Autodesk Fusion 360 part; units mm, degrees
(part 14 of 24)
  arc A3558 (64.6096, 1.6002) -> (64.6096, 1.5494) centre (64.6096, 1.5748) ccw
  arc A3559 (65.1035, 1.8344) -> (65.1543, 1.8344) centre (65.1289, 1.8344) ccw
  line L1262 (63.0301, 1.5748) -> (62.381, 1.5748)
  arc A3560 (61.588, 2.7432) -> (61.5372, 2.7432) centre (61.5626, 2.7432) ccw
  arc A3561 (60.071, 1.8994) -> (60.1218, 1.8994) centre (60.0964, 1.8994) ccw
  arc A3562 (62.7214, 2.763) -> (62.6897, 2.7234) centre (62.7055, 2.7432) ccw
  arc A3563 (65.9384, 2.7178) -> (65.9384, 2.7686) centre (65.9384, 2.7432) ccw
  line L1263 (64.6096, 1.5748) -> (64.8693, 1.5748)
  arc A3564 (65.5814, 1.8344) -> (65.841, 1.5748) centre (65.841, 1.8344) ccw
  arc A3565 (66.1727, 2.4836) -> (66.2235, 2.4836) centre (66.1981, 2.4836) ccw
  arc A3566 (60.1218, 2.7432) -> (60.071, 2.7432) centre (60.0964, 2.7432) ccw
  arc A3567 (65.6068, 1.8344) -> (65.556, 1.8344) centre (65.5814, 1.8344) ccw
  arc A3568 (64.8693, 1.6002) -> (64.8693, 1.5494) centre (64.8693, 1.5748) ccw
  arc A3569 (65.7112, 2.0616) -> (65.5814, 1.8344) centre (65.8451, 1.8344) ccw
  arc A3570 (66.96, 2.7432) -> (66.9092, 2.7432) centre (66.9346, 2.7432) ccw
  arc A3571 (66.6101, 2.7686) -> (66.6101, 2.7178) centre (66.6101, 2.7432) ccw
  line L1264 (67.2592, 2.7432) -> (66.6101, 2.7432)
  arc A3572 (65.841, 1.5494) -> (65.841, 1.6002) centre (65.841, 1.5748) ccw
  arc A3573 (62.6802, 1.5748) -> (62.731, 1.5748) centre (62.7056, 1.5748) ccw
  line L1265 (63.0301, 2.4836) -> (62.7056, 2.7432)
  arc A3574 (61.8712, 2.4637) -> (61.903, 2.5034) centre (61.8871, 2.4835) ccw
  arc A3575 (67.2592, 2.7178) -> (67.2592, 2.7686) centre (67.2592, 2.7432) ccw
  arc A3576 (65.1035, 2.4836) -> (65.1543, 2.4836) centre (65.1289, 2.4836) ccw
  arc A3577 (64.8693, 1.5494) -> (64.8693, 1.6002) centre (64.8693, 1.5748) ccw
  line L1266 (62.7056, 2.7432) -> (62.7056, 1.5748)
  arc A3578 (65.841, 1.6002) -> (65.841, 1.5494) centre (65.841, 1.5748) ccw
  arc A3579 (66.9092, 1.5748) -> (66.96, 1.5748) centre (66.9346, 1.5748) ccw
  arc A3580 (59.4473, 1.8994) -> (60.0964, 1.8994) centre (59.7719, 1.8994) ccw
  line L1267 (64.1731, 2.4836) -> (63.8486, 2.7432)
  arc A3581 (65.7241, 2.0397) -> (65.6983, 2.0835) centre (65.7112, 2.0616) ccw
  line L1268 (61.8871, 1.5748) -> (61.238, 1.5748)
  arc A3582 (65.6991, 2.0839) -> (65.7234, 2.0393) centre (65.7113, 2.0616) ccw
  line L1269 (63.8486, 2.7432) -> (63.8486, 1.5748)
  arc A3583 (62.731, 2.7432) -> (62.6802, 2.7432) centre (62.7056, 2.7432) ccw
  arc A3584 (65.841, 1.5748) -> (66.2305, 1.7371) centre (65.841, 2.1233) ccw
  arc A3585 (60.1218, 1.8994) -> (60.071, 1.8994) centre (60.0964, 1.8994) ccw
  arc A3586 (64.6096, 2.7686) -> (64.6096, 2.7178) centre (64.6096, 2.7432) ccw
  line L1270 (66.9346, 1.5748) -> (66.9346, 2.7432)
  arc A3587 (64.8693, 2.7686) -> (64.8693, 2.7178) centre (64.8693, 2.7432) ccw
  arc A3588 (63.874, 2.7432) -> (63.8232, 2.7432) centre (63.8486, 2.7432) ccw
  arc A3589 (59.4727, 1.8994) -> (59.4219, 1.8994) centre (59.4473, 1.8994) ccw
  arc A3590 (39.4305, 29.7091) -> (39.7238, 29.8306) centre (39.5772, 29.7698) ccw
  line L1271 (38.7475, 29.511) -> (39.41, 30.1735)
  line L1272 (52.2496, 23.4133) -> (52.3555, 23.3074)
  line L1273 (53.2211, 22.9489) -> (53.34, 22.9489)
  arc A3591 (53.1962, 22.7921) -> (53.2459, 23.1057) centre (53.2211, 22.9489) ccw
  arc A3592 (52.6878, 22.9182) -> (52.8319, 23.2011) centre (52.7599, 23.0597) ccw
  arc A3593 (47.9089, 22.8537) -> (47.9089, 22.5361) centre (47.9089, 22.6949) ccw
  line L1274 (28.1196, 27.3867) -> (27.813, 27.6933)
  arc A3594 (53.34, 22.7902) -> (53.34, 23.1077) centre (53.34, 22.9489) ccw
  arc A3595 (47.1478, 22.8514) -> (47.3723, 23.0759) centre (47.2601, 22.9636) ccw
  line L1275 (45.5255, 24.4221) -> (46.4947, 24.4221)
  line L1276 (52.9861, 22.9861) -> (53.2211, 22.9489)
  arc A3596 (52.4488, 23.4359) -> (52.2621, 23.179) centre (52.3555, 23.3075) ccw
  arc A3597 (52.2432, 23.1952) -> (52.4677, 23.4197) centre (52.3555, 23.3075) ccw
  arc A3598 (53.0109, 23.1429) -> (52.9613, 22.8293) centre (52.9861, 22.9861) ccw
  arc A3599 (47.3208, 23.1103) -> (47.1993, 22.817) centre (47.2601, 22.9636) ccw
  arc A3600 (47.8481, 22.5482) -> (47.9696, 22.8416) centre (47.9089, 22.6949) ccw
  arc A3601 (39.6894, 29.8821) -> (39.4649, 29.6576) centre (39.5772, 29.7699) ccw
  arc A3602 (52.62, 23.3091) -> (52.4758, 23.0262) centre (52.5479, 23.1677) ccw
  arc A3603 (29.3289, 27.6923) -> (29.3289, 28.0098) centre (29.3289, 27.8511) ccw
  arc A3604 (27.9717, 28.7366) -> (27.6542, 28.7366) centre (27.813, 28.7366) ccw
  arc A3605 (40.3906, 29.3851) -> (40.3906, 29.0676) centre (40.3906, 29.2264) ccw
  line L1277 (49.26, 22.9637) -> (49.53, 23.2337)
  line L1278 (46.4947, 24.4221) -> (46.4947, 24.1091)
  arc A3606 (52.3619, 23.301) -> (52.1373, 23.5255) centre (52.2496, 23.4133) ccw
  arc A3607 (52.8089, 23.2106) -> (52.7108, 22.9086) centre (52.7599, 23.0596) ccw
  arc A3608 (49.8608, 23.1103) -> (49.7393, 22.817) centre (49.8, 22.9637) ccw
  arc A3609 (29.0911, 28.0098) -> (29.0911, 27.6923) centre (29.0911, 27.8511) ccw
  line L1279 (39.9298, 29.4172) -> (40.3906, 29.2263)
  arc A3610 (39.5566, 30.2343) -> (39.2633, 30.1128) centre (39.41, 30.1736) ccw
  line L1280 (29.3289, 27.8511) -> (29.21, 27.8511)
  arc A3611 (50.4489, 22.8537) -> (50.4489, 22.5361) centre (50.4489, 22.6949) ccw
  arc A3612 (52.937, 22.8351) -> (53.0352, 23.1371) centre (52.9861, 22.9861) ccw
  arc A3613 (38.2666, 29.4837) -> (38.3881, 29.1903) centre (38.3274, 29.337) ccw
  line L1281 (46.7634, 23.4602) -> (47.26, 22.9637)
  line L1282 (51.8, 22.9637) -> (52.2496, 23.4133)
  line L1283 (52.7599, 23.0596) -> (52.9861, 22.9861)
  arc A3614 (51.0904, 22.8416) -> (51.2119, 22.5482) centre (51.1512, 22.6949) ccw
  line L1284 (52.5479, 23.1676) -> (52.7599, 23.0596)
  line L1285 (52.3555, 23.3074) -> (52.5479, 23.1676)
  arc A3615 (52.4546, 23.0392) -> (52.6412, 23.296) centre (52.5479, 23.1676) ccw
  line L1286 (40.5107, 29.2263) -> (45.1661, 24.571)
  line L1287 (49.8, 22.9637) -> (50.4489, 22.6949)
  arc A3616 (45.4647, 24.2754) -> (45.5862, 24.5688) centre (45.5255, 24.4221) ccw
  arc A3617 (46.6414, 24.1698) -> (46.348, 24.0483) centre (46.4947, 24.1091) ccw
  line L1288 (40.3906, 29.2263) -> (40.5107, 29.2263)
  arc A3618 (29.3538, 28.0079) -> (29.3041, 27.6943) centre (29.329, 27.8511) ccw
  line L1289 (53.34, 22.9489) -> (53.34, 25.4)
  arc A3619 (52.3619, 23.5255) -> (52.1373, 23.301) centre (52.2496, 23.4132) ccw
  arc A3620 (51.6877, 23.0759) -> (51.9122, 22.8514) centre (51.7999, 22.9637) ccw
  arc A3621 (49.1477, 23.0759) -> (49.3722, 22.8514) centre (49.26, 22.9637) ccw
  arc A3622 (40.5107, 29.0676) -> (40.5107, 29.3851) centre (40.5107, 29.2264) ccw
  arc A3623 (46.8757, 23.5725) -> (46.6512, 23.348) centre (46.7635, 23.4603) ccw
  arc A3624 (53.2211, 23.1077) -> (53.2211, 22.7902) centre (53.2211, 22.9489) ccw
  line L1290 (47.26, 22.9637) -> (47.9089, 22.6949)
  arc A3625 (45.2268, 24.7176) -> (45.1053, 24.4243) centre (45.166, 24.5709) ccw
  arc A3626 (51.8607, 22.817) -> (51.7392, 23.1103) centre (51.7999, 22.9637) ccw
  arc A3627 (48.6111, 22.5361) -> (48.6111, 22.8537) centre (48.6111, 22.6949) ccw
  arc A3628 (46.4947, 24.2633) -> (46.4947, 24.5809) centre (46.4947, 24.4221) ccw
  arc A3629 (45.5255, 24.5809) -> (45.5255, 24.2633) centre (45.5255, 24.4221) ccw
  arc A3630 (49.3207, 22.817) -> (49.1992, 23.1103) centre (49.26, 22.9637) ccw
  line L1291 (46.4947, 24.1091) -> (46.7634, 23.4602)
  arc A3631 (48.5504, 22.8416) -> (48.6719, 22.5482) centre (48.6112, 22.6949) ccw
  arc A3632 (45.0538, 24.4587) -> (45.2783, 24.6832) centre (45.166, 24.571) ccw
  line L1292 (48.6111, 22.6949) -> (49.26, 22.9637)
  arc A3633 (53.4988, 25.4) -> (53.1813, 25.4) centre (53.3401, 25.4) ccw
  line L1293 (49.53, 23.2337) -> (49.8, 22.9637)
  arc A3634 (53.1813, 22.9489) -> (53.4988, 22.9489) centre (53.3401, 22.9489) ccw
  line L1294 (54.7406, 23.8801) -> (54.8141, 24.1063)
  arc A3635 (53.4987, 25.4) -> (53.1812, 25.4) centre (53.34, 25.4) ccw
  arc A3636 (54.761, 23.5748) -> (54.5041, 23.7614) centre (54.6326, 23.6681) ccw
  arc A3637 (54.8513, 25.2413) -> (54.8513, 25.5588) centre (54.8513, 25.4001) ccw
  line L1295 (50.4489, 22.6949) -> (51.1511, 22.6949)
  arc A3638 (51.1511, 22.5361) -> (51.1511, 22.8537) centre (51.1511, 22.6949) ccw
  line L1296 (51.1511, 22.6949) -> (51.8, 22.9637)
  arc A3639 (46.336, 24.1091) -> (46.6534, 24.1091) centre (46.4947, 24.1091) ccw
  line L1297 (54.6326, 23.6681) -> (54.7406, 23.8801)
  line L1298 (54.1321, 23.1676) -> (54.3245, 23.3074)
  arc A3640 (53.34, 23.1077) -> (53.34, 22.7902) centre (53.34, 22.9489) ccw
  arc A3641 (46.6168, 23.3995) -> (46.9101, 23.521) centre (46.7634, 23.4603) ccw
  arc A3642 (54.6631, 26.6446) -> (54.9651, 26.7428) centre (54.8141, 26.6937) ccw
  line L1299 (54.4928, 23.4757) -> (54.6326, 23.6681)
  line L1300 (53.4589, 22.9489) -> (53.6939, 22.9861)
  arc A3643 (54.882, 23.808) -> (54.5991, 23.9521) centre (54.7405, 23.8801) ccw
  line L1301 (47.9089, 22.6949) -> (48.6111, 22.6949)
  arc A3644 (50.3881, 22.5482) -> (50.5096, 22.8416) centre (50.4489, 22.6949) ccw
  arc A3645 (54.2042, 23.0262) -> (54.06, 23.3091) centre (54.1321, 23.1677) ccw
  arc A3646 (49.6878, 22.8514) -> (49.9123, 23.0759) centre (49.8, 22.9637) ccw
  arc A3647 (55.0081, 24.3164) -> (54.6945, 24.3661) centre (54.8513, 24.3413) ccw
  arc A3648 (54.8513, 25.2412) -> (54.8513, 25.5587) centre (54.8513, 25.4) ccw
  line L1302 (53.34, 25.4) -> (54.8513, 25.4)
  arc A3649 (54.6945, 26.4339) -> (55.0081, 26.4836) centre (54.8513, 26.4588) ccw
  arc A3650 (46.6534, 24.4221) -> (46.336, 24.4221) centre (46.4947, 24.4221) ccw
  arc A3651 (49.6423, 23.1214) -> (49.4177, 23.3459) centre (49.53, 23.2336) ccw
  line L1303 (54.8141, 26.6937) -> (54.7406, 26.9199)
  arc A3652 (53.4341, 23.1057) -> (53.4838, 22.7921) centre (53.459, 22.9489) ccw
  arc A3653 (54.6925, 24.3413) -> (55.01, 24.3413) centre (54.8513, 24.3413) ccw
  line L1304 (54.8513, 25.4) -> (54.8513, 26.4587)
  arc A3654 (53.7187, 22.8293) -> (53.6691, 23.1429) centre (53.6939, 22.9861) ccw
  line L1305 (54.8513, 26.4587) -> (54.8141, 26.6937)
  arc A3655 (53.4589, 22.7902) -> (53.4589, 23.1077) centre (53.4589, 22.9489) ccw
  arc A3656 (54.5041, 27.0386) -> (54.761, 27.2252) centre (54.6326, 27.1319) ccw
  line L1306 (53.34, 25.4) -> (53.34, 22.9489)
  arc A3657 (54.9651, 24.0572) -> (54.6631, 24.1554) centre (54.8141, 24.1063) ccw
  arc A3658 (53.1813, 25.4) -> (53.4988, 25.4) centre (53.3401, 25.4) ccw
  arc A3659 (55.01, 26.4587) -> (54.6925, 26.4587) centre (54.8513, 26.4587) ccw
  arc A3660 (53.9692, 22.9086) -> (53.8711, 23.2106) centre (53.9201, 23.0596) ccw
  arc A3661 (49.6423, 23.3459) -> (49.4177, 23.1214) centre (49.53, 23.2336) ccw
  line L1307 (54.8513, 25.4) -> (53.34, 25.4)
  line L1308 (54.8141, 24.1063) -> (54.8513, 24.3413)
  line L1309 (54.4928, 27.3243) -> (54.3245, 27.4926)
  arc A3662 (53.34, 25.2412) -> (53.34, 25.5587) centre (53.34, 25.4) ccw
  line L1310 (54.7406, 26.9199) -> (54.6326, 27.1319)
  arc A3663 (54.9709, 26.7185) -> (54.6573, 26.6689) centre (54.8141, 26.6937) ccw
  arc A3664 (53.34, 25.5588) -> (53.34, 25.2413) centre (53.34, 25.4001) ccw
  line L1311 (54.8513, 24.3413) -> (54.8513, 25.4)
  line L1312 (45.1661, 24.571) -> (45.5255, 24.4221)
  arc A3665 (55.01, 25.4) -> (54.6925, 25.4) centre (54.8513, 25.4) ccw
  arc A3666 (40.623, 29.3386) -> (40.3985, 29.114) centre (40.5108, 29.2263) ccw
  arc A3667 (53.6448, 23.1371) -> (53.743, 22.8351) centre (53.6939, 22.9861) ccw
  arc A3668 (54.6212, 27.4177) -> (54.3643, 27.231) centre (54.4928, 27.3244) ccw
  arc A3669 (54.4179, 23.179) -> (54.2312, 23.4359) centre (54.3246, 23.3075) ccw
  arc A3670 (54.605, 23.3634) -> (54.3805, 23.5879) centre (54.4928, 23.4757) ccw
  arc A3671 (54.3643, 23.569) -> (54.6212, 23.3823) centre (54.4928, 23.4757) ccw
  arc A3672 (54.5896, 23.9291) -> (54.8916, 23.831) centre (54.7406, 23.8801) ccw
  arc A3673 (53.8481, 23.2011) -> (53.9922, 22.9182) centre (53.9202, 23.0597) ccw
  arc A3674 (52.9613, 27.9707) -> (53.0109, 27.6571) centre (52.9861, 27.8139) ccw
  arc A3675 (53.1812, 25.4) -> (53.4987, 25.4) centre (53.34, 25.4) ccw
  arc A3676 (54.6573, 24.1311) -> (54.9709, 24.0815) centre (54.8141, 24.1063) ccw
  arc A3677 (54.774, 27.204) -> (54.4911, 27.0598) centre (54.6326, 27.1319) ccw
  arc A3678 (54.5991, 26.8479) -> (54.882, 26.992) centre (54.7405, 26.92) ccw
  arc A3679 (53.34, 25.5587) -> (53.34, 25.2412) centre (53.34, 25.4) ccw
  arc A3680 (54.0388, 23.296) -> (54.2254, 23.0392) centre (54.1321, 23.1676) ccw
  line L1313 (53.34, 22.9489) -> (53.4589, 22.9489)
  arc A3681 (54.4911, 23.7402) -> (54.774, 23.596) centre (54.6326, 23.6681) ccw
  arc A3682 (54.8916, 26.969) -> (54.5896, 26.8709) centre (54.7406, 26.92) ccw
  arc A3683 (47.2781, 34.3097) -> (47.1566, 34.0163) centre (47.2174, 34.163) ccw
  arc A3684 (47.5767, 33.8423) -> (47.6982, 34.1357) centre (47.6375, 33.989) ccw
  arc A3685 (53.743, 27.9649) -> (53.6448, 27.6629) centre (53.6939, 27.8139) ccw
  arc A3686 (47.8467, 33.5552) -> (48.0712, 33.7797) centre (47.959, 33.6675) ccw
  arc A3687 (54.06, 27.4909) -> (54.2042, 27.7738) centre (54.1321, 27.6324) ccw
  line L1314 (52.9861, 27.8139) -> (52.7599, 27.7404)
  arc A3688 (53.34, 25.5587) -> (53.34, 25.2412) centre (53.34, 25.4) ccw
  arc A3689 (53.6691, 27.6571) -> (53.7187, 27.9707) centre (53.6939, 27.8139) ccw
  arc A3690 (53.0352, 27.6629) -> (52.937, 27.9649) centre (52.9861, 27.8139) ccw
  line L1315 (54.3245, 23.3074) -> (54.4928, 23.4757)
  arc A3691 (53.4988, 27.8511) -> (53.1813, 27.8511) centre (53.3401, 27.8511) ccw
  arc A3692 (51.6567, 29.7452) -> (51.8812, 29.9697) centre (51.769, 29.8575) ccw
  line L1316 (54.3245, 27.4926) -> (54.1321, 27.6324)
  arc A3693 (52.1017, 29.4374) -> (51.7842, 29.4374) centre (51.943, 29.4374) ccw
  line L1317 (53.34, 25.4) -> (53.34, 27.8511)
  arc A3694 (52.4677, 27.3803) -> (52.2432, 27.6048) centre (52.3555, 27.4926) ccw
  arc A3695 (53.4589, 27.6923) -> (53.4589, 28.0098) centre (53.4589, 27.8511) ccw
  arc A3696 (53.2459, 27.6943) -> (53.1962, 28.0079) centre (53.221, 27.8511) ccw
  arc A3697 (53.1812, 22.9489) -> (53.4987, 22.9489) centre (53.34, 22.9489) ccw
  arc A3698 (53.4987, 27.8511) -> (53.1812, 27.8511) centre (53.34, 27.8511) ccw
  line L1318 (53.9201, 27.7404) -> (53.6939, 27.8139)
  arc A3699 (51.7963, 29.3766) -> (52.0897, 29.4981) centre (51.943, 29.4374) ccw
  arc A3700 (53.2211, 28.0098) -> (53.2211, 27.6923) centre (53.2211, 27.8511) ccw
  arc A3701 (52.4758, 27.7738) -> (52.62, 27.4909) centre (52.5479, 27.6323) ccw
  arc A3702 (54.2123, 23.4197) -> (54.4368, 23.1952) centre (54.3246, 23.3075) ccw
  arc A3703 (54.6925, 25.4) -> (55.01, 25.4) centre (54.8513, 25.4) ccw
  arc A3704 (51.7842, 27.6933) -> (52.1017, 27.6933) centre (51.943, 27.6933) ccw
  line L1319 (53.9201, 23.0596) -> (54.1321, 23.1676)
  arc A3705 (53.1813, 25.4) -> (53.4988, 25.4) centre (53.3401, 25.4) ccw
  arc A3706 (53.8711, 27.5894) -> (53.9692, 27.8914) centre (53.9202, 27.7404) ccw
  arc A3707 (53.34, 25.5588) -> (53.34, 25.2413) centre (53.34, 25.4001) ccw
  arc A3708 (54.2312, 27.3641) -> (54.4179, 27.621) centre (54.3246, 27.4925) ccw
  arc A3709 (52.6412, 27.5039) -> (52.4546, 27.7608) centre (52.5479, 27.6324) ccw
  line L1320 (53.2211, 27.8511) -> (52.9861, 27.8139)
  arc A3710 (52.8319, 27.5989) -> (52.6878, 27.8818) centre (52.7599, 27.7404) ccw
  line L1321 (52.5479, 27.6324) -> (52.3555, 27.4926)
  arc A3711 (53.9922, 27.8818) -> (53.8481, 27.5989) centre (53.9202, 27.7403) ccw
  line L1322 (54.6326, 27.1319) -> (54.4928, 27.3243)
  arc A3712 (53.34, 28.0098) -> (53.34, 27.6923) centre (53.34, 27.8511) ccw
  line L1323 (53.34, 27.8511) -> (53.34, 25.4)
  line L1324 (53.6939, 22.9861) -> (53.9201, 23.0596)
  arc A3713 (54.4368, 27.6048) -> (54.2123, 27.3803) centre (54.3246, 27.4925) ccw
  line L1325 (53.6939, 27.8139) -> (53.4589, 27.8511)
  arc A3714 (53.4988, 25.4) -> (53.1813, 25.4) centre (53.3401, 25.4) ccw
  arc A3715 (22.9777, 29.0302) -> (23.2022, 28.8056) centre (23.09, 28.9179) ccw
  arc A3716 (9.7155, 29.0766) -> (9.7155, 28.7591) centre (9.7155, 28.9179) ccw
  arc A3717 (41.5984, 34.3217) -> (41.5984, 34.0042) centre (41.5984, 34.163) ccw
  arc A3718 (40.1368, 34.3936) -> (39.9123, 34.6182) centre (40.0246, 34.5059) ccw
  arc A3719 (51.5597, 30.2912) -> (51.3352, 30.0667) centre (51.4475, 30.179) ccw
  arc A3720 (52.7108, 27.8914) -> (52.8089, 27.5894) centre (52.7599, 27.7404) ccw
  arc A3721 (54.2254, 27.7608) -> (54.0388, 27.5039) centre (54.1321, 27.6323) ccw
  line L1326 (40.0245, 34.5059) -> (39.1541, 33.6355)
  line L1327 (23.5113, 29.3393) -> (23.0899, 28.9179)
  arc A3722 (39.2664, 33.0383) -> (39.0418, 33.2628) centre (39.1541, 33.1506) ccw
  arc A3723 (27.0833, 31.0152) -> (26.8588, 31.2397) centre (26.9711, 31.1275) ccw
  arc A3724 (47.7497, 34.1012) -> (47.5252, 33.8767) centre (47.6375, 33.9889) ccw
  arc A3725 (25.5874, 30.3851) -> (25.3629, 30.1606) centre (25.4751, 30.2728) ccw
  line L1328 (23.5113, 29.4594) -> (23.5113, 29.3393)
  arc A3726 (37.6266, 31.4642) -> (37.6266, 31.7817) centre (37.6266, 31.623) ccw
  line L1329 (47.2174, 34.163) -> (41.5984, 34.163)
  arc A3727 (41.3677, 34.6181) -> (41.1432, 34.3936) centre (41.2555, 34.5058) ccw
  line L1330 (25.7958, 29.9522) -> (25.4752, 30.2728)
  line L1331 (27.7126, 31.623) -> (27.2925, 31.449)
  arc A3728 (41.2555, 34.3471) -> (41.2555, 34.6646) centre (41.2555, 34.5058) ccw
  arc A3729 (38.9954, 33.1505) -> (39.3128, 33.1505) centre (39.1541, 33.1505) ccw
  arc A3730 (27.2318, 31.5957) -> (27.3533, 31.3023) centre (27.2926, 31.449) ccw
  line L1332 (26.971, 31.1275) -> (26.0225, 30.179)
  arc A3731 (53.4838, 28.0079) -> (53.4341, 27.6943) centre (53.459, 27.8511) ccw
  arc A3732 (39.3128, 33.6355) -> (38.9954, 33.6355) centre (39.1541, 33.6355) ccw
  arc A3733 (40.0245, 34.6646) -> (40.0245, 34.3471) centre (40.0245, 34.5058) ccw
  arc A3734 (51.3352, 30.0667) -> (51.5597, 30.2912) centre (51.4475, 30.179) ccw
  arc A3735 (52.2621, 27.621) -> (52.4488, 27.3641) centre (52.3555, 27.4925) ccw
  arc A3736 (25.6835, 30.0645) -> (25.908, 29.84) centre (25.7958, 29.9522) ccw
  arc A3737 (51.9157, 29.9182) -> (51.6223, 29.7967) centre (51.769, 29.8575) ccw
  line L1333 (51.943, 29.4374) -> (51.769, 29.8575)
  arc A3738 (48.0712, 33.7797) -> (47.8467, 33.5552) centre (47.959, 33.6675) ccw
  line L1334 (23.0899, 28.9179) -> (9.7155, 28.9179)
  line L1335 (39.1541, 33.1505) -> (37.6266, 31.623)
  arc A3739 (23.8488, 29.8594) -> (23.5555, 29.9809) centre (23.7022, 29.9202) ccw
  line L1336 (52.3555, 27.4926) -> (52.2496, 27.3867)
  arc A3740 (54.3805, 27.2121) -> (54.605, 27.4366) centre (54.4928, 27.3244) ccw
  line L1337 (51.4475, 30.179) -> (47.959, 33.6675)
  line L1338 (47.959, 33.6675) -> (47.6375, 33.989)
  line L1339 (26.0225, 30.179) -> (25.7958, 29.9522)
  line L1340 (41.2555, 34.5059) -> (40.0245, 34.5059)
  arc A3741 (23.6236, 29.227) -> (23.399, 29.4515) centre (23.5113, 29.3393) ccw
  arc A3742 (23.0899, 28.7591) -> (23.0899, 29.0766) centre (23.0899, 28.9179) ccw
  line L1341 (54.1321, 27.6324) -> (53.9201, 27.7404)
  arc A3743 (53.34, 25.2413) -> (53.34, 25.5588) centre (53.34, 25.4001) ccw
  arc A3744 (52.0553, 27.8056) -> (51.8307, 27.5811) centre (51.943, 27.6934) ccw
  line L1342 (52.2496, 27.3867) -> (51.943, 27.6933)
  line L1343 (51.943, 27.6933) -> (51.943, 29.4374)
  line L1344 (51.769, 29.8575) -> (51.4475, 30.179)
  arc A3745 (52.1373, 27.499) -> (52.3619, 27.2744) centre (52.2496, 27.3867) ccw
  arc A3746 (52.1373, 27.2744) -> (52.3619, 27.499) centre (52.2496, 27.3867) ccw
  line L1345 (53.4589, 27.8511) -> (53.34, 27.8511)
  arc A3747 (53.34, 27.6923) -> (53.34, 28.0098) centre (53.34, 27.8511) ccw
  line L1346 (53.34, 27.8511) -> (53.2211, 27.8511)
  line L1347 (52.7599, 27.7404) -> (52.5479, 27.6324)
  line L1348 (47.6375, 33.989) -> (47.2174, 34.163)
  arc A3748 (25.4144, 30.1262) -> (25.5359, 30.4195) centre (25.4752, 30.2728) ccw
  line L1349 (70.3249, 35.8521) -> (70.4098, 35.7672)
  arc A3749 (71.9424, 38.0051) -> (71.7179, 37.7806) centre (71.8302, 37.8928) ccw
  arc A3750 (23.5899, 30.0324) -> (23.8144, 29.8079) centre (23.7021, 29.9202) ccw
  line L1350 (25.0144, 30.4637) -> (24.5156, 30.4637)
  line L1351 (41.5984, 34.163) -> (41.2555, 34.5059)
  arc A3751 (27.7734, 31.4763) -> (27.6519, 31.7697) centre (27.7127, 31.623) ccw
  line L1352 (23.7022, 29.9202) -> (23.5113, 29.4594)
  arc A3752 (26.0225, 30.3377) -> (26.0225, 30.0202) centre (26.0225, 30.179) ccw
  arc A3753 (26.1348, 30.0667) -> (25.9103, 30.2912) centre (26.0225, 30.179) ccw
  arc A3754 (41.4861, 34.0507) -> (41.7106, 34.2752) centre (41.5984, 34.1629) ccw
  arc A3755 (27.1298, 31.1275) -> (26.8123, 31.1275) centre (26.9711, 31.1275) ccw
  arc A3756 (24.5764, 30.317) -> (24.4549, 30.6104) centre (24.5157, 30.4637) ccw
  arc A3757 (72.3295, 37.6009) -> (72.0362, 37.4794) centre (72.1829, 37.5401) ccw
  line L1353 (70.8706, 38.0837) -> (70.4098, 37.8928)
  arc A3758 (70.3491, 38.0395) -> (70.4706, 37.7462) centre (70.4099, 37.8929) ccw
  line L1354 (70.4098, 37.8928) -> (70.3249, 37.8079)
  line L1355 (24.5156, 30.4637) -> (24.0548, 30.2728)
  line L1356 (24.0548, 30.2728) -> (23.7022, 29.9202)
  arc A3759 (53.9953, 37.8057) -> (54.1168, 37.5124) centre (54.0561, 37.6591) ccw
  arc A3760 (54.1683, 37.5468) -> (53.9438, 37.7713) centre (54.0561, 37.6591) ccw
  arc A3761 (26.0225, 30.0202) -> (26.0225, 30.3377) centre (26.0225, 30.179) ccw
  arc A3762 (70.8706, 38.2424) -> (70.8706, 37.9249) centre (70.8706, 38.0837) ccw
  arc A3763 (27.7126, 31.7817) -> (27.7126, 31.4642) centre (27.7126, 31.623) ccw
  arc A3764 (25.6835, 29.84) -> (25.908, 30.0645) centre (25.7958, 29.9522) ccw
  arc A3765 (23.3646, 29.5201) -> (23.658, 29.3986) centre (23.5113, 29.4593) ccw
  arc A3766 (47.2174, 34.0042) -> (47.2174, 34.3217) centre (47.2174, 34.163) ccw
  arc A3767 (26.8123, 31.1275) -> (27.1298, 31.1275) centre (26.9711, 31.1275) ccw
  line L1357 (39.1541, 33.6355) -> (39.1541, 33.1505)
  arc A3768 (25.9103, 30.2912) -> (26.1348, 30.0667) centre (26.0225, 30.179) ccw
  arc A3769 (23.6701, 29.4594) -> (23.3526, 29.4594) centre (23.5113, 29.4594) ccw
  arc A3770 (52.1271, 32.4045) -> (52.4446, 32.4045) centre (52.2858, 32.4045) ccw
  arc A3771 (70.9314, 37.937) -> (70.8099, 38.2304) centre (70.8707, 38.0837) ccw
  arc A3772 (72.5204, 36.5199) -> (72.227, 36.6414) centre (72.3737, 36.5806) ccw
  line L1358 (37.6266, 31.623) -> (27.7126, 31.623)
  line L1359 (27.2925, 31.449) -> (26.971, 31.1275)
  line L1360 (25.4752, 30.2728) -> (25.0144, 30.4637)
  arc A3773 (25.0751, 30.6104) -> (24.9536, 30.317) centre (25.0144, 30.4637) ccw
  arc A3774 (70.2126, 37.9202) -> (70.4372, 37.6956) centre (70.3249, 37.8079) ccw
  arc A3775 (72.0362, 36.1806) -> (72.3295, 36.0591) centre (72.1829, 36.1198) ccw
  arc A3776 (72.5324, 37.0794) -> (72.2149, 37.0794) centre (72.3736, 37.0794) ccw
  arc A3777 (72.227, 37.0186) -> (72.5204, 37.1401) centre (72.3737, 37.0793) ccw
  arc A3778 (37.5143, 31.7353) -> (37.7388, 31.5107) centre (37.6266, 31.623) ccw
  arc A3779 (9.5567, 28.9179) -> (9.8742, 28.9179) centre (9.7155, 28.9179) ccw
  line L1361 (54.4155, 37.8079) -> (54.0561, 37.659)
  line L1362 (71.8302, 37.8928) -> (71.3694, 38.0837)
  arc A3780 (27.4048, 31.3367) -> (27.1803, 31.5612) centre (27.2926, 31.449) ccw
  line L1363 (53.781, 37.3839) -> (50.9029, 34.5059)
  arc A3781 (26.8588, 31.2397) -> (27.0833, 31.0152) centre (26.9711, 31.1275) ccw
  line L1364 (9.7155, 28.9179) -> (9.7155, 30.078)
  arc A3782 (54.4155, 37.9666) -> (54.4155, 37.6491) centre (54.4155, 37.8079) ccw
  arc A3783 (24.5156, 30.6224) -> (24.5156, 30.3049) centre (24.5156, 30.4637) ccw
  line L1365 (70.3249, 37.8079) -> (54.4155, 37.8079)
  arc A3784 (23.9941, 30.4195) -> (24.1156, 30.1262) centre (24.0549, 30.2728) ccw
  arc A3785 (39.0418, 33.7477) -> (39.2664, 33.5232) centre (39.1541, 33.6355) ccw
  line L1366 (72.1828, 36.1198) -> (72.3737, 36.5806)
  arc A3786 (70.4706, 35.9138) -> (70.3491, 35.6205) centre (70.4099, 35.7672) ccw
  arc A3787 (72.2149, 36.5806) -> (72.5324, 36.5806) centre (72.3736, 36.5806) ccw
  arc A3788 (24.1671, 30.1606) -> (23.9426, 30.3851) centre (24.0548, 30.2728) ccw
  arc A3789 (23.3526, 29.3393) -> (23.6701, 29.3393) centre (23.5113, 29.3393) ccw
  arc A3790 (25.0144, 30.3049) -> (25.0144, 30.6224) centre (25.0144, 30.4637) ccw
  arc A3791 (54.4762, 37.6612) -> (54.3547, 37.9546) centre (54.4155, 37.8079) ccw
  arc A3792 (72.517, 13.1763) -> (72.517, 13.4938) centre (72.517, 13.335) ccw
  arc A3793 (5.9114, 14.1288) -> (5.9114, 13.8113) centre (5.9114, 13.9701) ccw
  arc A3794 (84.2253, 13.8113) -> (84.2253, 14.1288) centre (84.2253, 13.9701) ccw
  arc A3795 (10.273, 14.1288) -> (10.273, 13.8113) centre (10.273, 13.9701) ccw
  arc A3796 (83.8894, 13.4938) -> (83.8894, 13.1763) centre (83.8894, 13.335) ccw
  arc A3797 (75.452, 11.9063) -> (75.452, 12.2238) centre (75.452, 12.0651) ccw
  arc A3798 (44.4663, 13.8113) -> (44.4663, 14.1288) centre (44.4663, 13.9701) ccw
  arc A3799 (16.7064, 14.7637) -> (16.7064, 14.4463) centre (16.7064, 14.605) ccw
  arc A3800 (72.517, 13.4938) -> (72.517, 13.1763) centre (72.517, 13.335) ccw
  arc A3801 (82.282, 14.1288) -> (82.282, 13.8113) centre (82.282, 13.9701) ccw
  arc A3802 (13.7736, 14.4463) -> (13.7736, 14.7637) centre (13.7736, 14.605) ccw
  arc A3803 (0.7747, 14.7637) -> (0.7747, 14.4463) centre (0.7747, 14.605) ccw
  arc A3804 (14.4467, 12.5413) -> (14.4467, 12.8588) centre (14.4467, 12.7001) ccw
  arc A3805 (84.2253, 13.1763) -> (84.2253, 13.4938) centre (84.2253, 13.335) ccw
  arc A3806 (79.488, 13.4938) -> (79.488, 13.1763) centre (79.488, 13.335) ccw
  arc A3807 (47.512, 14.4463) -> (47.512, 14.7637) centre (47.512, 14.605) ccw
  arc A3808 (70.598, 12.8588) -> (70.598, 12.5413) centre (70.598, 12.7001) ccw
  arc A3809 (73.7489, 12.2238) -> (73.7489, 11.9063) centre (73.7489, 12.0651) ccw
  arc A3810 (71.2851, 11.9063) -> (71.2851, 12.2238) centre (71.2851, 12.0651) ccw
  arc A3811 (21.717, 14.4463) -> (21.717, 14.7637) centre (21.717, 14.605) ccw
  arc A3812 (84.2253, 12.5413) -> (84.2253, 12.8588) centre (84.2253, 12.7001) ccw
  arc A3813 (76.087, 12.5413) -> (76.087, 12.8588) centre (76.087, 12.7001) ccw
  arc A3814 (72.517, 11.9063) -> (72.517, 12.2238) centre (72.517, 12.0651) ccw
  arc A3815 (71.2851, 12.5413) -> (71.2851, 12.8588) centre (71.2851, 12.7001) ccw
  arc A3816 (46.814, 14.7637) -> (46.814, 14.4463) centre (46.814, 14.605) ccw
  arc A3817 (25.7464, 12.8588) -> (25.7464, 12.5413) centre (25.7464, 12.7001) ccw
  arc A3818 (44.7421, 11.9063) -> (44.7421, 12.2238) centre (44.7421, 12.0651) ccw
  arc A3819 (69.328, 14.1288) -> (69.328, 13.8113) centre (69.328, 13.9701) ccw
  arc A3820 (68.693, 14.7637) -> (68.693, 14.4463) centre (68.693, 14.605) ccw
  arc A3821 (46.6979, 12.2238) -> (46.6979, 11.9063) centre (46.6979, 12.0651) ccw
  arc A3822 (0.7747, 14.1288) -> (0.7747, 13.8113) centre (0.7747, 13.9701) ccw
  arc A3823 (8.142, 13.1763) -> (8.142, 13.4938) centre (8.142, 13.335) ccw
  arc A3824 (11.543, 12.8588) -> (11.543, 12.5413) centre (11.543, 12.7001) ccw
  arc A3825 (72.517, 12.5413) -> (72.517, 12.8588) centre (72.517, 12.7001) ccw
  arc A3826 (46.6979, 12.8588) -> (46.6979, 12.5413) centre (46.6979, 12.7001) ccw
  arc A3827 (81.1911, 12.5413) -> (81.1911, 12.8588) centre (81.1911, 12.7001) ccw
  arc A3828 (71.233, 12.2238) -> (71.233, 11.9063) centre (71.233, 12.0651) ccw
  arc A3829 (67.832, 12.5413) -> (67.832, 12.8588) centre (67.832, 12.7001) ccw
  arc A3830 (4.2867, 12.5413) -> (4.2867, 12.8588) centre (4.2867, 12.7001) ccw
  arc A3831 (13.7541, 15.0813) -> (13.7541, 15.3987) centre (13.7541, 15.24) ccw
  arc A3832 (81.1911, 11.9063) -> (81.1911, 12.2238) centre (81.1911, 12.0651) ccw
  arc A3833 (9.003, 15.3987) -> (9.003, 15.0813) centre (9.003, 15.24) ccw
  arc A3834 (21.6335, 15.0813) -> (21.6335, 15.3987) centre (21.6335, 15.24) ccw
  arc A3835 (16.0714, 14.1288) -> (16.0714, 13.8113) centre (16.0714, 13.9701) ccw
  arc A3836 (3.6136, 14.4463) -> (3.6136, 14.7637) centre (3.6136, 14.605) ccw
  arc A3837 (21.2436, 13.8113) -> (21.2436, 14.1288) centre (21.2436, 13.9701) ccw
  arc A3838 (3.5941, 15.0813) -> (3.5941, 15.3987) centre (3.5941, 15.24) ccw
  arc A3839 (77.992, 14.4463) -> (77.992, 14.7637) centre (77.992, 14.605) ccw
  arc A3840 (24.4764, 14.1288) -> (24.4764, 13.8113) centre (24.4764, 13.9701) ccw
  arc A3841 (84.2253, 14.4463) -> (84.2253, 14.7637) centre (84.2253, 14.605) ccw
  arc A3842 (84.2253, 15.7163) -> (84.2253, 16.0338) centre (84.2253, 15.875) ccw
  arc A3843 (3.6136, 15.7163) -> (3.6136, 16.0338) centre (3.6136, 15.875) ccw
  arc A3844 (14.4086, 13.8113) -> (14.4086, 14.1288) centre (14.4086, 13.9701) ccw
  arc A3845 (13.7736, 15.7163) -> (13.7736, 16.0338) centre (13.7736, 15.875) ccw
  arc A3846 (26.7135, 15.0813) -> (26.7135, 15.3987) centre (26.7135, 15.24) ccw
  arc A3847 (49.008, 16.0338) -> (49.008, 15.7163) centre (49.008, 15.875) ccw
  arc A3848 (68.404, 16.0338) -> (68.404, 15.7163) centre (68.404, 15.875) ccw
  arc A3849 (34.2465, 15.3987) -> (34.2465, 15.0813) centre (34.2465, 15.24) ccw
  arc A3850 (46.9737, 14.1288) -> (46.9737, 13.8113) centre (46.9737, 13.9701) ccw
  arc A3851 (24.003, 14.7637) -> (24.003, 14.4463) centre (24.003, 14.605) ccw
  arc A3852 (39.8168, 15.0813) -> (39.8168, 15.3987) centre (39.8168, 15.24) ccw
  arc A3853 (4.2486, 16.3513) -> (4.2486, 16.6688) centre (4.2486, 16.51) ccw
  arc A3854 (0.7747, 16.6688) -> (0.7747, 16.3513) centre (0.7747, 16.51) ccw
  arc A3855 (77.357, 13.8113) -> (77.357, 14.1288) centre (77.357, 13.9701) ccw
  arc A3856 (44.626, 14.4463) -> (44.626, 14.7637) centre (44.626, 14.605) ccw
  arc A3857 (49.643, 15.3987) -> (49.643, 15.0813) centre (49.643, 15.24) ccw
  arc A3858 (83.4507, 15.3987) -> (83.4507, 15.0813) centre (83.4507, 15.24) ccw
  arc A3859 (7.507, 13.8113) -> (7.507, 14.1288) centre (7.507, 13.9701) ccw
  arc A3860 (36.8735, 15.0813) -> (36.8735, 15.3987) centre (36.8735, 15.24) ccw
  arc A3861 (8.368, 16.0338) -> (8.368, 15.7163) centre (8.368, 15.875) ccw
  arc A3862 (83.5279, 16.0338) -> (83.5279, 15.7163) centre (83.5279, 15.875) ccw
  arc A3863 (75.0912, 15.3987) -> (75.0912, 15.0813) centre (75.0912, 15.24) ccw
  arc A3864 (48.147, 13.8113) -> (48.147, 14.1288) centre (48.147, 13.9701) ccw
  arc A3865 (70.1386, 15.7163) -> (70.1386, 16.0338) centre (70.1386, 15.875) ccw
  arc A3866 (73.3702, 13.4938) -> (73.3702, 13.1763) centre (73.3702, 13.335) ccw
  arc A3867 (21.2123, 15.7163) -> (21.2123, 16.0338) centre (21.2123, 15.875) ccw
  arc A3868 (76.722, 13.1763) -> (76.722, 13.4938) centre (76.722, 13.335) ccw
  arc A3869 (82.917, 14.7637) -> (82.917, 14.4463) centre (82.917, 14.605) ccw
  arc A3870 (4.2486, 13.8113) -> (4.2486, 14.1288) centre (4.2486, 13.9701) ccw
  arc A3871 (9.638, 14.7637) -> (9.638, 14.4463) centre (9.638, 14.605) ccw
  arc A3872 (0.7747, 15.3987) -> (0.7747, 15.0813) centre (0.7747, 15.24) ccw
  arc A3873 (81.4646, 13.1763) -> (81.4646, 13.4938) centre (81.4646, 13.335) ccw
  arc A3874 (84.2253, 15.0813) -> (84.2253, 15.3987) centre (84.2253, 15.24) ccw
  arc A3875 (46.877, 15.0813) -> (46.877, 15.3987) centre (46.877, 15.24) ccw
  arc A3876 (40.64, 15.3987) -> (40.64, 15.0813) centre (40.64, 15.24) ccw
  arc A3877 (47.738, 17.3038) -> (47.738, 16.9862) centre (47.738, 17.145) ccw
  arc A3878 (0.7747, 17.9388) -> (0.7747, 17.6212) centre (0.7747, 17.78) ccw
  arc A3879 (31.7935, 17.6212) -> (31.7935, 17.9388) centre (31.7935, 17.78) ccw
  arc A3880 (36.7865, 15.3987) -> (36.7865, 15.0813) centre (36.7865, 15.24) ccw
  arc A3881 (83.5279, 16.6688) -> (83.5279, 16.3513) centre (83.5279, 16.51) ccw
  arc A3882 (40.64, 16.0338) -> (40.64, 15.7163) centre (40.64, 15.875) ccw
  arc A3883 (83.5279, 17.3038) -> (83.5279, 16.9862) centre (83.5279, 17.145) ccw
  arc A3884 (68.5637, 16.6688) -> (68.5637, 16.3513) centre (68.5637, 16.51) ccw
  arc A3885 (0.7747, 16.0338) -> (0.7747, 15.7163) centre (0.7747, 15.875) ccw
  arc A3886 (78.627, 15.0813) -> (78.627, 15.3987) centre (78.627, 15.24) ccw
  arc A3887 (31.7065, 17.9388) -> (31.7065, 17.6212) centre (31.7065, 17.78) ccw
  arc A3888 (34.3335, 15.0813) -> (34.3335, 15.3987) centre (34.3335, 15.24) ccw
  line L1367 (29.1665, 17.78) -> (29.2535, 17.78)
  arc A3889 (5.9114, 16.6688) -> (5.9114, 16.3513) centre (5.9114, 16.51) ccw
  arc A3890 (73.3464, 15.0813) -> (73.3464, 15.3987) centre (73.3464, 15.24) ccw
  arc A3891 (29.2535, 15.0813) -> (29.2535, 15.3987) centre (29.2535, 15.24) ccw
  arc A3892 (40.64, 15.0813) -> (40.64, 15.3987) centre (40.64, 15.24) ccw
  arc A3893 (16.7064, 16.0338) -> (16.7064, 15.7163) centre (16.7064, 15.875) ccw
  arc A3894 (48.373, 16.6688) -> (48.373, 16.3513) centre (48.373, 16.51) ccw
  arc A3895 (53.34, 17.3038) -> (53.34, 16.9862) centre (53.34, 17.145) ccw
  line L1368 (31.7065, 17.78) -> (31.7935, 17.78)
  arc A3896 (29.1665, 15.3987) -> (29.1665, 15.0813) centre (29.1665, 15.24) ccw
  arc A3897 (21.2123, 16.9862) -> (21.2123, 17.3038) centre (21.2123, 17.145) ccw
  arc A3898 (21.0947, 16.3513) -> (21.0947, 16.6688) centre (21.0947, 16.51) ccw
  line L1369 (34.2465, 17.78) -> (34.3335, 17.78)
  arc A3899 (34.3335, 17.6212) -> (34.3335, 17.9388) centre (34.3335, 17.78) ccw
  arc A3900 (46.242, 15.7163) -> (46.242, 16.0338) centre (46.242, 15.875) ccw
  arc A3901 (68.8685, 16.9862) -> (68.8685, 17.3038) centre (68.8685, 17.145) ccw
  arc A3902 (42.0126, 17.3038) -> (42.0126, 16.9862) centre (42.0126, 17.145) ccw
  arc A3903 (21.6335, 17.6212) -> (21.6335, 17.9388) centre (21.6335, 17.78) ccw
  arc A3904 (39.3265, 15.3987) -> (39.3265, 15.0813) centre (39.3265, 15.24) ccw
  arc A3905 (57.037, 16.3513) -> (57.037, 16.6688) centre (57.037, 16.51) ccw
  arc A3906 (26.6265, 17.9388) -> (26.6265, 17.6212) centre (26.6265, 17.78) ccw
  arc A3907 (40.64, 15.7163) -> (40.64, 16.0338) centre (40.64, 15.875) ccw
  line L1370 (26.6265, 17.78) -> (26.7135, 17.78)
  arc A3908 (24.1735, 15.0813) -> (24.1735, 15.3987) centre (24.1735, 15.24) ccw
  arc A3909 (53.34, 16.9862) -> (53.34, 17.3038) centre (53.34, 17.145) ccw
  arc A3910 (41.4632, 15.3987) -> (41.4632, 15.0813) centre (41.4632, 15.24) ccw
  arc A3911 (16.7259, 15.3987) -> (16.7259, 15.0813) centre (16.7259, 15.24) ccw
  arc A3912 (31.7935, 15.0813) -> (31.7935, 15.3987) centre (31.7935, 15.24) ccw
  arc A3913 (26.6265, 15.3987) -> (26.6265, 15.0813) centre (26.6265, 15.24) ccw
  arc A3914 (42.0126, 16.0338) -> (42.0126, 15.7163) centre (42.0126, 15.875) ccw
  arc A3915 (14.4086, 16.3513) -> (14.4086, 16.6688) centre (14.4086, 16.51) ccw
  arc A3916 (24.0865, 15.3987) -> (24.0865, 15.0813) centre (24.0865, 15.24) ccw
  arc A3917 (31.7065, 15.3987) -> (31.7065, 15.0813) centre (31.7065, 15.24) ccw
  arc A3918 (57.672, 15.7163) -> (57.672, 16.0338) centre (57.672, 15.875) ccw
  arc A3919 (51.9547, 16.6688) -> (51.9547, 16.3513) centre (51.9547, 16.51) ccw
  arc A3920 (84.2253, 16.3513) -> (84.2253, 16.6688) centre (84.2253, 16.51) ccw
  line L1371 (24.0865, 17.78) -> (24.1735, 17.78)
  arc A3921 (69.5036, 16.3513) -> (69.5036, 16.6688) centre (69.5036, 16.51) ccw
  arc A3922 (49.6453, 18.8912) -> (49.6453, 19.2088) centre (49.6453, 19.05) ccw
  arc A3923 (52.5445, 18.8912) -> (52.5445, 19.2088) centre (52.5445, 19.05) ccw
  arc A3924 (39.3265, 17.9388) -> (39.3265, 17.6212) centre (39.3265, 17.78) ccw
  arc A3925 (29.1665, 17.9388) -> (29.1665, 17.6212) centre (29.1665, 17.78) ccw
  arc A3926 (54.7705, 18.5738) -> (54.7705, 18.2562) centre (54.7705, 18.415) ccw
  arc A3927 (83.5279, 17.9388) -> (83.5279, 17.6212) centre (83.5279, 17.78) ccw
  arc A3928 (52.5445, 16.3513) -> (52.5445, 16.6688) centre (52.5445, 16.51) ccw
  arc A3929 (0.7747, 17.3038) -> (0.7747, 16.9862) centre (0.7747, 17.145) ccw
  arc A3930 (40.64, 16.6688) -> (40.64, 16.3513) centre (40.64, 16.51) ccw
  arc A3931 (45.607, 16.3513) -> (45.607, 16.6688) centre (45.607, 16.51) ccw
  arc A3932 (16.0714, 16.6688) -> (16.0714, 16.3513) centre (16.0714, 16.51) ccw
  arc A3933 (44.7421, 18.8912) -> (44.7421, 19.2088) centre (44.7421, 19.05) ccw
  arc A3934 (53.34, 16.3513) -> (53.34, 16.6688) centre (53.34, 16.51) ccw
  arc A3935 (44.972, 16.9862) -> (44.972, 17.3038) centre (44.972, 17.145) ccw
  arc A3936 (68.404, 17.3038) -> (68.404, 16.9862) centre (68.404, 17.145) ccw
  arc A3937 (53.34, 17.9388) -> (53.34, 17.6212) centre (53.34, 17.78) ccw
  arc A3938 (49.2073, 16.9862) -> (49.2073, 17.3038) centre (49.2073, 17.145) ccw
  arc A3939 (24.1735, 17.6212) -> (24.1735, 17.9388) centre (24.1735, 17.78) ccw
  arc A3940 (26.7135, 17.6212) -> (26.7135, 17.9388) centre (26.7135, 17.78) ccw
  arc A3941 (29.2535, 17.6212) -> (29.2535, 17.9388) centre (29.2535, 17.78) ccw
  arc A3942 (57.898, 18.5738) -> (57.898, 18.2562) centre (57.898, 18.415) ccw
  arc A3943 (73.5304, 18.2562) -> (73.5304, 18.5738) centre (73.5304, 18.415) ccw
  arc A3944 (68.2336, 17.6212) -> (68.2336, 17.9388) centre (68.2336, 17.78) ccw
  arc A3945 (49.6453, 16.3513) -> (49.6453, 16.6688) centre (49.6453, 16.51) ccw
  arc A3946 (84.2253, 16.9862) -> (84.2253, 17.3038) centre (84.2253, 17.145) ccw
  arc A3947 (70.8314, 18.5738) -> (70.8314, 18.2562) centre (70.8314, 18.415) ccw
  arc A3948 (46.6979, 19.2088) -> (46.6979, 18.8912) centre (46.6979, 19.05) ccw
  arc A3949 (53.34, 16.6688) -> (53.34, 16.3513) centre (53.34, 16.51) ccw
  arc A3950 (54.7705, 17.3038) -> (54.7705, 16.9862) centre (54.7705, 17.145) ccw
  arc A3951 (34.2465, 17.9388) -> (34.2465, 17.6212) centre (34.2465, 17.78) ccw
  arc A3952 (40.64, 16.9862) -> (40.64, 17.3038) centre (40.64, 17.145) ccw
  arc A3953 (56.402, 16.9862) -> (56.402, 17.3038) centre (56.402, 17.145) ccw
  arc A3954 (54.1355, 16.6688) -> (54.1355, 16.3513) centre (54.1355, 16.51) ccw
  arc A3955 (24.0865, 17.9388) -> (24.0865, 17.6212) centre (24.0865, 17.78) ccw
  arc A3956 (40.64, 17.3038) -> (40.64, 16.9862) centre (40.64, 17.145) ccw
  arc A3957 (80.0328, 18.2562) -> (80.0328, 18.5738) centre (80.0328, 18.415) ccw
  arc A3958 (0.7747, 19.2088) -> (0.7747, 18.8912) centre (0.7747, 19.05) ccw
  arc A3959 (51.9547, 19.2088) -> (51.9547, 18.8912) centre (51.9547, 19.05) ccw
  arc A3960 (55.767, 17.6212) -> (55.767, 17.9388) centre (55.767, 17.78) ccw
  line L1372 (57.263, 19.05) -> (57.5886, 19.05)
  arc A3961 (81.5721, 18.2562) -> (81.5721, 18.5738) centre (81.5721, 18.415) ccw
  arc A3962 (36.7865, 17.9388) -> (36.7865, 17.6212) centre (36.7865, 17.78) ccw
  arc A3963 (54.1355, 19.2088) -> (54.1355, 18.8912) centre (54.1355, 19.05) ccw
  arc A3964 (0.7747, 18.5738) -> (0.7747, 18.2562) centre (0.7747, 18.415) ccw
  arc A3965 (40.64, 17.6212) -> (40.64, 17.9388) centre (40.64, 17.78) ccw
  arc A3966 (83.5279, 19.8438) -> (83.5279, 19.5263) centre (83.5279, 19.6851) ccw
  arc A3967 (84.2253, 19.5263) -> (84.2253, 19.8438) centre (84.2253, 19.6851) ccw
  arc A3968 (40.64, 17.9388) -> (40.64, 17.6212) centre (40.64, 17.78) ccw
  line L1373 (39.3265, 17.78) -> (39.8168, 17.78)
  arc A3969 (56.9341, 20.1612) -> (56.9341, 20.4788) centre (56.9341, 20.32) ccw
  arc A3970 (70.1964, 20.4788) -> (70.1964, 20.1612) centre (70.1964, 20.32) ccw
  arc A3971 (44.7421, 20.1612) -> (44.7421, 20.4788) centre (44.7421, 20.32) ccw
  arc A3972 (6.2857, 20.1612) -> (6.2857, 20.4788) centre (6.2857, 20.32) ccw
  arc A3973 (36.8735, 17.6212) -> (36.8735, 17.9388) centre (36.8735, 17.78) ccw
  arc A3974 (83.5279, 18.5738) -> (83.5279, 18.2562) centre (83.5279, 18.415) ccw
  arc A3975 (44.7421, 18.2562) -> (44.7421, 18.5738) centre (44.7421, 18.415) ccw
  arc A3976 (41.4632, 17.9388) -> (41.4632, 17.6212) centre (41.4632, 17.78) ccw
  arc A3977 (79.2208, 20.1612) -> (79.2208, 20.4788) centre (79.2208, 20.32) ccw
  line L1374 (81.4096, 18.415) -> (81.5721, 18.415)
  arc A3978 (53.34, 18.5738) -> (53.34, 18.2562) centre (53.34, 18.415) ccw
  arc A3979 (72.7184, 20.1612) -> (72.7184, 20.4788) centre (72.7184, 20.32) ccw
  arc A3980 (84.2253, 20.1612) -> (84.2253, 20.4788) centre (84.2253, 20.32) ccw
  arc A3981 (8.9543, 20.4788) -> (8.9543, 20.1612) centre (8.9543, 20.32) ccw
  arc A3982 (46.6979, 18.5738) -> (46.6979, 18.2562) centre (46.6979, 18.415) ccw
  arc A3983 (75.7192, 20.4788) -> (75.7192, 20.1612) centre (75.7192, 20.32) ccw
  arc A3984 (59.2514, 19.2088) -> (59.2514, 18.8912) centre (59.2514, 19.05) ccw
  arc A3985 (83.3742, 20.4788) -> (83.3742, 20.1612) centre (83.3742, 20.32) ccw
  line L1375 (36.7865, 17.78) -> (36.8735, 17.78)
  arc A3986 (7.62, 20.1612) -> (7.62, 20.4788) centre (7.62, 20.32) ccw
  arc A3987 (39.8168, 17.6212) -> (39.8168, 17.9388) centre (39.8168, 17.78) ccw
  line L1376 (54.7705, 18.415) -> (55.132, 18.415)
  arc A3988 (53.34, 18.2562) -> (53.34, 18.5738) centre (53.34, 18.415) ccw
  arc A3989 (81.4096, 18.5738) -> (81.4096, 18.2562) centre (81.4096, 18.415) ccw
  arc A3990 (74.9072, 18.5738) -> (74.9072, 18.2562) centre (74.9072, 18.415) ccw
  arc A3991 (53.34, 19.2088) -> (53.34, 18.8912) centre (53.34, 19.05) ccw
  arc A3992 (44.7421, 17.6212) -> (44.7421, 17.9388) centre (44.7421, 17.78) ccw
  arc A3993 (47.103, 17.9388) -> (47.103, 17.6212) centre (47.103, 17.78) ccw
  arc A3994 (84.2253, 17.6212) -> (84.2253, 17.9388) centre (84.2253, 17.78) ccw
  arc A3995 (49.2073, 18.2562) -> (49.2073, 18.5738) centre (49.2073, 18.415) ccw
  arc A3996 (53.34, 18.8912) -> (53.34, 19.2088) centre (53.34, 19.05) ccw
  arc A3997 (49.0855, 17.6212) -> (49.0855, 17.9388) centre (49.0855, 17.78) ccw
  arc A3998 (54.9021, 18.8912) -> (54.9021, 19.2088) centre (54.9021, 19.05) ccw
  arc A3999 (58.533, 17.9388) -> (58.533, 17.6212) centre (58.533, 17.78) ccw
  arc A4000 (55.132, 18.2562) -> (55.132, 18.5738) centre (55.132, 18.415) ccw
  arc A4001 (67.6058, 18.2562) -> (67.6058, 18.5738) centre (67.6058, 18.415) ccw
  arc A4002 (84.2253, 18.2562) -> (84.2253, 18.5738) centre (84.2253, 18.415) ccw
  arc A4003 (0.7747, 21.1138) -> (0.7747, 20.7963) centre (0.7747, 20.955) ccw
  arc A4004 (7.62, 21.1138) -> (7.62, 20.7963) centre (7.62, 20.955) ccw
  arc A4005 (56.9536, 19.5263) -> (56.9536, 19.8438) centre (56.9536, 19.6851) ccw
  arc A4006 (7.62, 20.4788) -> (7.62, 20.1612) centre (7.62, 20.32) ccw
  arc A4007 (57.5886, 18.8912) -> (57.5886, 19.2088) centre (57.5886, 19.05) ccw
  arc A4008 (57.263, 19.2088) -> (57.263, 18.8912) centre (57.263, 19.05) ccw
  arc A4009 (83.5279, 19.2088) -> (83.5279, 18.8912) centre (83.5279, 19.05) ccw
  arc A4010 (5.7785, 20.7963) -> (5.7785, 21.1138) centre (5.7785, 20.955) ccw
  arc A4011 (7.62, 20.7963) -> (7.62, 21.1138) centre (7.62, 20.955) ccw
  arc A4012 (84.2253, 18.8912) -> (84.2253, 19.2088) centre (84.2253, 19.05) ccw
  arc A4013 (74.9072, 19.8438) -> (74.9072, 19.5263) centre (74.9072, 19.6851) ccw
  arc A4014 (0.7747, 19.8438) -> (0.7747, 19.5263) centre (0.7747, 19.6851) ccw
  arc A4015 (46.6979, 20.4788) -> (46.6979, 20.1612) centre (46.6979, 20.32) ccw
  line L1377 (56.8579, 20.32) -> (56.9341, 20.32)
  arc A4016 (56.8579, 20.4788) -> (56.8579, 20.1612) centre (56.8579, 20.32) ccw
  arc A4017 (67.0941, 20.1612) -> (67.0941, 20.4788) centre (67.0941, 20.32) ccw
  arc A4018 (59.9059, 20.4788) -> (59.9059, 20.1612) centre (59.9059, 20.32) ccw
  arc A4019 (0.7747, 20.4788) -> (0.7747, 20.1612) centre (0.7747, 20.32) ccw
  arc A4020 (46.6979, 19.8438) -> (46.6979, 19.5263) centre (46.6979, 19.6851) ccw
  arc A4021 (54.9021, 19.5263) -> (54.9021, 19.8438) centre (54.9021, 19.6851) ccw
  arc A4022 (71.4591, 21.7488) -> (71.4591, 21.4312) centre (71.4591, 21.59) ccw
  arc A4023 (84.2253, 21.4312) -> (84.2253, 21.7488) centre (84.2253, 21.59) ccw
  arc A4024 (44.7421, 19.5263) -> (44.7421, 19.8438) centre (44.7421, 19.6851) ccw
  arc A4025 (81.5721, 18.8912) -> (81.5721, 19.2088) centre (81.5721, 19.05) ccw
  arc A4026 (7.62, 22.0663) -> (7.62, 22.3838) centre (7.62, 22.2251) ccw
  arc A4027 (7.62, 22.3838) -> (7.62, 22.0663) centre (7.62, 22.2251) ccw
  arc A4028 (56.8579, 21.7488) -> (56.8579, 21.4312) centre (56.8579, 21.59) ccw
  line L1378 (56.8579, 19.685) -> (56.9536, 19.685)
  line L1379 (56.8579, 20.955) -> (56.9536, 20.955)
  arc A4029 (56.8579, 19.8438) -> (56.8579, 19.5263) centre (56.8579, 19.6851) ccw
  arc A4030 (44.464, 20.7963) -> (44.464, 21.1138) centre (44.464, 20.955) ccw
  arc A4031 (43.194, 22.0663) -> (43.194, 22.3838) centre (43.194, 22.2251) ccw
  arc A4032 (70.0464, 19.8438) -> (70.0464, 19.5263) centre (70.0464, 19.6851) ccw
  arc A4033 (70.1964, 19.2088) -> (70.1964, 18.8912) centre (70.1964, 19.05) ccw
  arc A4034 (67.437, 18.8912) -> (67.437, 19.2088) centre (67.437, 19.05) ccw
  arc A4035 (54.9021, 20.1612) -> (54.9021, 20.4788) centre (54.9021, 20.32) ccw
  arc A4036 (59.8864, 19.8438) -> (59.8864, 19.5263) centre (59.8864, 19.6851) ccw
  arc A4037 (80.0328, 19.5263) -> (80.0328, 19.8438) centre (80.0328, 19.6851) ccw
  arc A4038 (59.2514, 21.7488) -> (59.2514, 21.4312) centre (59.2514, 21.59) ccw
  arc A4039 (73.5304, 19.5263) -> (73.5304, 19.8438) centre (73.5304, 19.6851) ccw
  arc A4040 (72.4535, 21.4312) -> (72.4535, 21.7488) centre (72.4535, 21.59) ccw
  arc A4041 (67.1136, 19.5263) -> (67.1136, 19.8438) centre (67.1136, 19.6851) ccw
  arc A4042 (5.7785, 22.0663) -> (5.7785, 22.3838) centre (5.7785, 22.2251) ccw
  arc A4043 (48.9268, 17.439) -> (49.2443, 17.439) centre (49.0856, 17.439) ccw
  line L1380 (53.34, 17.78) -> (53.34, 16.3195)
  line L1381 (51.7712, 16.3265) -> (52.2496, 16.8049)
  arc A4044 (54.6417, 17.175) -> (54.9592, 17.175) centre (54.8005, 17.175) ccw
  arc A4045 (57.5886, 21.4312) -> (57.5886, 21.7488) centre (57.5886, 21.59) ccw
  arc A4046 (82.7392, 21.1138) -> (82.7392, 20.7963) centre (82.7392, 20.955) ccw
  arc A4047 (53.1813, 17.78) -> (53.4988, 17.78) centre (53.3401, 17.78) ccw
  arc A4048 (45.96, 22.3838) -> (45.96, 22.0663) centre (45.96, 22.2251) ccw
  arc A4049 (54.9021, 22.0663) -> (54.9021, 22.3838) centre (54.9021, 22.2251) ccw
  arc A4050 (53.34, 17.9387) -> (53.34, 17.6212) centre (53.34, 17.78) ccw
  arc A4051 (54.9021, 20.7963) -> (54.9021, 21.1138) centre (54.9021, 20.955) ccw
  arc A4052 (48.9388, 18.1818) -> (49.2322, 18.0603) centre (49.0855, 18.1211) ccw
  line L1382 (54.8005, 17.175) -> (54.8005, 17.78)
  arc A4053 (53.4987, 17.78) -> (53.1812, 17.78) centre (53.34, 17.78) ccw
  arc A4054 (56.8579, 21.1138) -> (56.8579, 20.7963) centre (56.8579, 20.955) ccw
  arc A4055 (72.4553, 20.7963) -> (72.4553, 21.1138) centre (72.4553, 20.955) ccw
  arc A4056 (54.9592, 18.385) -> (54.6417, 18.385) centre (54.8005, 18.385) ccw
  line L1383 (54.8005, 18.385) -> (53.945, 19.2405)
  line L1384 (49.8288, 19.2335) -> (49.3465, 18.7512)
  arc A4057 (0.7747, 22.3838) -> (0.7747, 22.0663) centre (0.7747, 22.2251) ccw
  line L1385 (54.8005, 17.78) -> (53.34, 17.78)
  line L1386 (54.8005, 17.78) -> (54.8005, 18.385)
  arc A4058 (51.6589, 16.4388) -> (51.8834, 16.2143) centre (51.7712, 16.3266) ccw
  line L1387 (53.34, 16.3195) -> (53.945, 16.3195)
  arc A4059 (46.6979, 21.1138) -> (46.6979, 20.7963) centre (46.6979, 20.955) ccw
  arc A4060 (53.1813, 16.3195) -> (53.4988, 16.3195) centre (53.3401, 16.3195) ccw
  arc A4061 (51.141, 15.9068) -> (51.141, 16.2243) centre (51.141, 16.0655) ccw
  line L1388 (52.2496, 16.8049) -> (52.735, 16.3195)
  arc A4062 (53.945, 16.1608) -> (53.945, 16.4783) centre (53.945, 16.3195) ccw
  arc A4063 (82.663, 21.7488) -> (82.663, 21.4312) centre (82.663, 21.59) ccw
  arc A4064 (7.62, 21.7488) -> (7.62, 21.4312) centre (7.62, 21.59) ccw
  arc A4065 (54.9021, 21.4312) -> (54.9021, 21.7488) centre (54.9021, 21.59) ccw
  arc A4066 (67.1136, 20.7963) -> (67.1136, 21.1138) centre (67.1136, 20.955) ccw
  arc A4067 (56.9536, 20.7963) -> (56.9536, 21.1138) centre (56.9536, 20.955) ccw
  arc A4068 (54.0572, 19.3528) -> (53.8327, 19.1282) centre (53.945, 19.2405) ccw
  arc A4069 (70.8314, 21.1138) -> (70.8314, 20.7963) centre (70.8314, 20.955) ccw
  line L1389 (53.945, 19.2405) -> (53.34, 19.2405)
  arc A4070 (67.7486, 21.4312) -> (67.7486, 21.7488) centre (67.7486, 21.59) ccw
  arc A4071 (52.6228, 16.2072) -> (52.8473, 16.4318) centre (52.7351, 16.3195) ccw
  arc A4072 (54.8005, 17.6213) -> (54.8005, 17.9388) centre (54.8005, 17.78) ccw
  arc A4073 (9.4615, 22.3838) -> (9.4615, 22.0663) centre (9.4615, 22.2251) ccw
  line L1390 (53.34, 17.78) -> (54.8005, 17.78)
  arc A4074 (46.3862, 22.0233) -> (46.1617, 21.7988) centre (46.2739, 21.9111) ccw
  arc A4075 (84.2253, 20.7963) -> (84.2253, 21.1138) centre (84.2253, 20.955) ccw
  arc A4076 (9.4615, 21.1138) -> (9.4615, 20.7963) centre (9.4615, 20.955) ccw
  arc A4077 (0.7747, 21.7488) -> (0.7747, 21.4312) centre (0.7747, 21.59) ccw
  arc A4078 (43.829, 21.4312) -> (43.829, 21.7488) centre (43.829, 21.59) ccw
  arc A4079 (46.568, 21.7488) -> (46.568, 21.4312) centre (46.568, 21.59) ccw
  arc A4080 (49.4932, 18.6904) -> (49.1998, 18.8119) centre (49.3465, 18.7512) ccw
  arc A4081 (53.34, 17.9388) -> (53.34, 17.6213) centre (53.34, 17.78) ccw
  line L1391 (46.2739, 21.911) -> (43.1258, 25.0591)
  arc A4082 (7.62, 21.4312) -> (7.62, 21.7488) centre (7.62, 21.59) ccw
  arc A4083 (59.8864, 21.1138) -> (59.8864, 20.7963) centre (59.8864, 20.955) ccw
  arc A4084 (54.6417, 17.78) -> (54.9592, 17.78) centre (54.8005, 17.78) ccw
  arc A4085 (12.1476, 33.5781) -> (12.465, 33.5781) centre (12.3063, 33.5781) ccw
  line L1392 (51.141, 16.0655) -> (51.7712, 16.3265)
  arc A4086 (49.1998, 16.7481) -> (49.4932, 16.8696) centre (49.3465, 16.8088) ccw
  arc A4087 (49.9411, 19.1212) -> (49.7166, 19.3457) centre (49.8288, 19.2335) ccw
  line L1393 (49.3465, 16.8088) -> (49.8288, 16.3265)
  arc A4088 (52.3619, 16.9172) -> (52.1374, 16.6927) centre (52.2497, 16.8049) ccw
  line L1394 (53.945, 16.3195) -> (54.8005, 17.175)
  arc A4089 (53.34, 16.4783) -> (53.34, 16.1608) centre (53.34, 16.3195) ccw